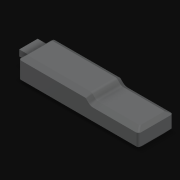
# Autodesk Inventor part: V5 Simple Battery
Saved by Autodesk Inventor 2021 (Build 250183000, 183)
## iProperties
Created: 2020-05-27
Part Number: V5 Simple Battery
Material: Generic
Document SubType Name: Modeling
Designer: Charlie Grier
Density: 1 g/cm^3
Appearance: Default
Author: Charlie Grier
Autodesk Inventor part; units mm, degrees
ref_plane "YZ Plane" through (0, 0, 0) normal (1, 0, 0) x (0, 1, 0)
ref_plane "XZ Plane" through (0, 0, 0) normal (0, 1, 0) x (-1, 0, 0)
ref_plane "XY Plane" through (0, 0, 0) normal (0, 0, 1) x (1, 0, 0)
sketch "Sketch1" plane through (0, 0, 0) normal (0, 0, 1) x (1, 0, 0)
  line L0 (0, 0) -> (160.4518, 0)
  line L1 (160.4518, 0) -> (160.4518, 30.4038)
  line L2 (160.4518, 30.4038) -> (0, 30.4038)
  line L3 (0, 30.4038) -> (0, 0)
  line L4 (97.5982, 24.1046) -> (160.4518, 24.1046)
  line L5 (95.9612, 25.7556) -> (92.9894, 28.7528) construction
  line L6 (91.3524, 30.4038) -> (97.5982, 24.1046)
  dimension "d0" = 160.4518
  dimension "d1" = 30.4038
  dimension "d4" = 67.4624
  dimension "d5" = 1.651
  dimension "d8" = 64.4906
  dimension "d9" = 4.6482
  dimension "d10" = 6.2992
  constraints: 14 end point, 4 point on line, 2 parallel, 2 perpendicular, 1 horizontal
  measures "d0" distance of L2.end L1.end
  measures "d1" distance of L1.end L0.end
  measures "d4" distance from line of L1 L5.end
  measures "d5" distance from line of L2 L5.end
  measures "d8" distance from line of L1 L5.start
  measures "d9" distance from line of L2 L5.start
  measures "d10" distance between parallel lines of L2 L4
extrude "Extrusion1" add sketch "Sketch1" along normal blind 46.4312 contours L3 L2 L6 L4 L1 L0
fillet "Fillet1" radius 5.6642 2 edges at (91.3524, 30.4038, 23.2156) (97.5982, 24.1046, 23.2156)
chamfer "Chamfer1" distance 4.5974 distance2 4.0894 1 edges at (160.4518, 24.1046, 23.2156) measured on face at (140.2874, 24.1046, 15.4771)
chamfer "Chamfer3" distance 4.0894 distance2 6.4516 3 edges at (127.9065, 24.1046, 0) (94.4753, 27.2542, 0) (44.496, 30.4038, 0) measured on face at (86.4331, 8.0715, 0)
chamfer "Chamfer2" distance 4.0894 distance2 6.4516 3 edges at (127.9065, 24.1046, 46.4312) (94.4753, 27.2542, 46.4312) (44.496, 30.4038, 46.4312) measured on face at (86.4331, 8.0715, 46.4312)
chamfer "Chamfer4" distance 4.0894 distance2 4.5974 1 edges at (0, 30.4038, 23.2156) measured on face at (0, 10.1346, 28.8036)
chamfer "Chamfer5" distance 3.429 distance2 4.0132 1 edges at (0, 0, 23.2156) measured on face at (0, 17.5429, 30.9541)
chamfer "Chamfer6" distance 3.8862 distance2 6.3246 1 edges at (82.2325, 0, 46.4312) measured on face at (87.5035, 6.7349, 46.4312)
chamfer "Chamfer7" distance 4.0132 distance2 3.429 1 edges at (160.4518, 0, 20.0533) measured on face at (160.4518, 13.3435, 28.8459)
chamfer "Chamfer8" distance 3.8862 distance2 6.3246 1 edges at (80.518, 0, 0) measured on face at (86.3605, 6.7349, 0)
fillet "Fillet2" radius 3.175 12 edges at (0, 15.1003, 0) (2.2987, 28.3591, 3.2258) (0, 15.1003, 46.4312) (2.2987, 28.3591, 43.2054) (2.0066, 1.7145, 3.5343) (2.0066, 1.7145, 42.8969) (158.683, 1.9431, 3.1623) (160.4518, 12.0142, 0) (158.1531, 22.0599, 3.2258) (158.1531, 22.0599, 43.2054) (160.4518, 12.0142, 46.4312) (158.683, 1.9431, 43.2689)
sketch "Sketch2" plane through (0, 3.429, 43.2562) normal (-1, 0, 0) x (0, 0, 1)
  line L0 (-32.0153, 0.1) -> (-56.6979, 0.1) construction
  line L1 (-56.6979, 0.1) -> (-56.6979, 8.3256) construction
  line L2 (-56.6979, 8.3256) -> (-32.0153, 8.3256) construction
  line L3 (-32.0153, 8.3256) -> (-32.0153, 0.1) construction
  ellipse E0 centre (-40.1387, 8.5022) end of major axis (-39.8909, 8.2522) minor radius 0.0031 (-40.1387, 8.4978) -> (-39.8909, 8.2522) ccw construction
  line L4 (-48.8131, 12.2136) -> (-39.9668, 12.2136) construction
  line L5 (-39.9668, 12.2136) -> (-39.9668, 8.3256) construction
  line L6 (-39.9668, 8.3256) -> (-48.8131, 8.3256) construction
  line L7 (-48.8131, 8.3256) -> (-48.8131, 12.2136) construction
  line L8 (-38.1, 18.161) -> (-13.4174, 18.161)
  line L9 (-13.4174, 18.161) -> (-13.4174, 9.9354)
  line L10 (-13.4174, 9.9354) -> (-38.1, 9.9354)
  line L11 (-38.1, 9.9354) -> (-38.1, 18.161)
  line L12 (-30.2152, 9.9354) -> (-21.3689, 9.9354)
  line L13 (-21.3689, 9.9354) -> (-21.3689, 6.0474)
  line L14 (-21.3689, 6.0474) -> (-30.2152, 6.0474)
  line L15 (-30.2152, 6.0474) -> (-30.2152, 9.9354)
  line L16 (-5.4645, 26.9748) -> (-34.6167, 26.9748) projected
  line L17 (-43.2562, 22.8854) -> (-43.2562, 0.4572) projected
  point P0 (-43.2562, -3.429)
  point P1 (-21.3689, 9.9354)
  dimension "d40" = 8.8464
  dimension "d41" = 8.2256
  dimension "d42" = 24.6826
  dimension "d43" = 3.888
  dimension "d44" = 7.8848
  dimension "d45" = 8.2256
  dimension "d46" = 24.6826
  dimension "d47" = 7.8848
  dimension "d48" = 3.888
  dimension "d49" = 8.8464
  dimension "d50" = 7.9515
  dimension "d51" = 7.9515
  dimension "d52" = 8.8138
  dimension "d53" = 5.1562
  constraints: 32 end point, 8 parallel, 4 horizontal, 4 perpendicular, 2 point on line, 5 other
  measures "d40" distance of L4.start L4.end
  measures "d41" distance of L0.end L1.end
  measures "d42" distance of L0.start L0.end
  measures "d43" distance of L6.end L4.start
  measures "d44" distance between parallel lines of L1 L7
  measures "d45" distance of L10.end L8.start
  measures "d46" distance of L9.end L10.end
  measures "d47" distance between parallel lines of L11 L15
  measures "d48" distance of L14.end L12.start
  measures "d49" distance of L13.end L14.end
  measures "d50" distance between parallel lines of L3 L5
  measures "d51" distance between parallel lines of L9 L13
  measures "d52" distance between parallel lines of L16 L8
  measures "d53" distance between parallel lines of L17 L11
extrude "Extrusion2" add sketch "Sketch2" along normal blind 15.875
equation "\"d45\" = d41"
equation "\"d46\" = d42"
equation "\"d47\" = d44"
equation "\"d48\" = d43"
equation "\"d49\" = d40"
body "Solid1"
